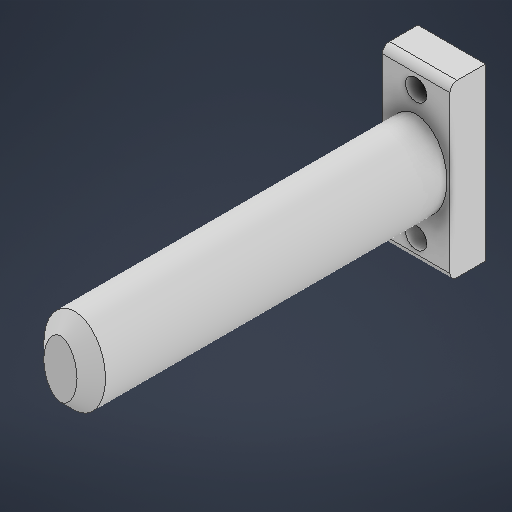
# Autodesk Inventor part: apoioP
Saved by Autodesk Inventor 2026 (Build 300175050, 175E)
## iProperties
Created: 2025-06-10
Part Number: apoioP
Material: Generic
Document SubType Name: Modeling
Designer: dcana
Density: 1 g/cm^3
Appearance: Default
Author: dcana
Autodesk Inventor part; units mm, degrees
ref_plane "YZ Plane" through (0, 0, 0) normal (1, 0, 0) x (0, 1, 0)
ref_plane "XZ Plane" through (0, 0, 0) normal (0, 1, 0) x (-1, 0, 0)
ref_plane "XY Plane" through (0, 0, 0) normal (0, 0, 1) x (1, 0, 0)
sketch "Sketch1" plane through (0, 0, 0) normal (0, 0, 1) x (1, 0, 0)
  line L0 (0, 0) -> (8.5363, 0)
  circle A0 centre (0, 9) radius 1.5
  circle A1 centre (0, -9) radius 1.5
  line L1 (-4.7525, 12.0011) -> (4.7525, 12.0011)
  line L2 (4.7525, 12.0011) -> (4.7525, -12.0011)
  line L3 (4.7525, -12.0011) -> (-4.7525, -12.0011)
  line L4 (-4.7525, -12.0011) -> (-4.7525, 12.0011)
  ellipse E0 centre (0, 0) end of major axis (0, 6.027) minor radius 4.3359
  ellipse E1 centre (-34.059, -8.6397) end of major axis (-34.059, -4.9131) minor radius 2.5528
  ellipse E2 centre (-34.1113, -8.6921) end of major axis (-34.1113, -2.6651) minor radius 4.3359
  point P0 (0, 12.0011)
  point P1 (0, -12.0011)
  point P2 (-4.7525, 0)
  point P3 (4.7525, 0)
  constraints: 10 end point, 4 midpoint, 2 centre point, 2 horizontal, 2 parallel, 1 coincident, 1 perpendicular, 6 other
extrude "Extrusion1" add sketch "Sketch1" along normal blind 5 contours L2 L3 L4 L1
sketch "Sketch2" plane through (0, 0, 5) normal (0, 0, 1) x (1, 0, 0)
  point P0 (0, 0)
sketch "Sketch3" plane through (0, 0, 5) normal (0, 0, 1) x (1, 0, 0)
  ellipse E0 centre (0, 0) end of major axis (0, -6.027) minor radius 4.3359 projected
  constraints: 1 other
extrude "Extrusion2" add sketch "Sketch3" along normal blind 50 and the other way blind 5
chamfer "Chamfer1" distance 2 angle 45 1 edges at (0, 6.027, 55)
fillet "Fillet1" radius 1 1 edges at (0, 12.0011, 5)
fillet "Fillet2" radius 1 1 edges at (0, -12.0011, 5)
body "Solid1"
